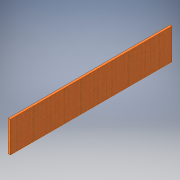
# Autodesk Inventor part: Home Depot Composite Slat 34 in
Saved by Autodesk Inventor 2016 (Build 200138000, 138)
## iProperties
Created: 2015-05-30
Part Number: Home Depot Composite Slat 34 in
Material: Wood (Cherry)
Document SubType Name: Modeling
Designer: steele
Density: 0.63 g/cm^3
Appearance: Cherry - Natural Low Gloss
Author: steele
Autodesk Inventor part; units mm, degrees
ref_plane "YZ Plane" through (0, 0, 0) normal (1, 0, 0) x (0, 1, 0)
ref_plane "XZ Plane" through (0, 0, 0) normal (0, 1, 0) x (-1, 0, 0)
ref_plane "XY Plane" through (0, 0, 0) normal (0, 0, 1) x (1, 0, 0)
sketch "Sketch1" plane through (0, 0, 0) normal (1, 0, 0) x (0, 1, 0)
  line L0 (-82.55, 431.8) -> (-82.55, -431.8)
  line L1 (-82.55, -431.8) -> (82.55, -431.8)
  line L2 (82.55, -431.8) -> (82.55, 431.8)
  line L3 (82.55, 431.8) -> (-82.55, 431.8)
  line L4 (-82.55, 431.8) -> (82.55, -431.8) construction
  line L5 (-82.55, -431.8) -> (82.55, 431.8) construction
  point P0 (0, 0)
  dimension "d0" = 863.6
  dimension "d1" = 165.1
  constraints: 12 end point, 2 midpoint, 2 parallel, 1 perpendicular, 1 vertical
  measures "d0" distance of L1.end L2.end
  measures "d1" distance of L0.end L1.end
extrude "Extrusion1" add sketch "Sketch1" along normal blind 11.1125
body "Solid1"
